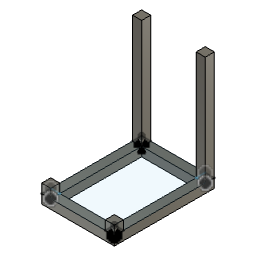
phone holder (Autodesk Fusion 360 design; units mm, degrees)
Autodesk Fusion 360 part; units mm, degrees
sketch "Sketch1" plane through (0, 0, 0) normal (0, 0, 1) x (1, 0, 0)
  line L0 (0, 0) -> (40, 0)
  line L1 (40, 0) -> (40, 55)
  line L2 (40, 55) -> (0, 55)
  line L3 (0, 55) -> (0, 0)
  line L4 (5, 5) -> (35, 5)
  line L5 (35, 5) -> (35, 50)
  line L6 (35, 50) -> (5, 50)
  line L7 (5, 50) -> (5, 5)
  dimension "d1" = 40
  dimension "d2" = 55
  dimension "d3" = 30
  dimension "d4" = 45
  constraint horizontal L0
  constraint vertical L1
  constraint horizontal L2
  constraint vertical L3
  constraint coincident L0.start L3.end
  constraint horizontal L4
  constraint vertical L5
  constraint horizontal L6
  constraint vertical L7
  measures "d1" distance of L0.start L0.end
  measures "d2" distance of L0.start L2.end
  measures "d3" distance of L4.start L4.end
  measures "d4" distance of L4.start L6.end
extrude "Extrude1" add sketch "Sketch1" along normal blind 5
sketch "Sketch2" plane through (0, 0, 5) normal (0, 0, 1) x (-1, 0, 0)
  line L0 (-5, -5) -> (-5, -50)
  line L1 (-5, -50) -> (-35, -50)
  line L2 (-35, -50) -> (-35, -5)
  line L3 (-35, -5) -> (-5, -5)
  line L4 (0, -55) -> (0, 0)
  line L5 (0, 0) -> (-40, 0)
  line L6 (-40, 0) -> (-40, -55)
  line L7 (-40, -55) -> (0, -55)
  line L8 (0, -55) -> (-5, -55)
  line L9 (-5, -55) -> (-5, -50)
  line L10 (-5, -50) -> (0, -50)
  line L11 (0, -50) -> (0, -55)
  line L12 (-35, -55) -> (-40, -55)
  line L13 (-40, -55) -> (-40, -50)
  line L14 (-40, -50) -> (-35, -50)
  line L15 (-35, -50) -> (-35, -55)
  line L16 (-35, -5) -> (-40, -5)
  line L17 (-40, -5) -> (-40, 0)
  line L18 (-40, 0) -> (-35, 0)
  line L19 (-35, 0) -> (-35, -5)
  line L20 (0, -5) -> (-5, -5)
  line L21 (-5, -5) -> (-5, 0)
  line L22 (-5, 0) -> (0, 0)
  line L23 (0, 0) -> (0, -5)
  constraint horizontal L8
  constraint vertical L9
  constraint horizontal L10
  constraint vertical L11
  constraint coincident L0.end L1.start
  constraint coincident L4.start L7.end
  constraint horizontal L12
  constraint vertical L13
  constraint horizontal L14
  constraint vertical L15
  constraint coincident L6 L13.end
  constraint coincident L7 L12.start
  constraint horizontal L16
  constraint vertical L17
  constraint horizontal L18
  constraint vertical L19
  constraint coincident L5.end L6.start
  constraint coincident L2.end L3.start
  constraint horizontal L20
  constraint vertical L21
  constraint horizontal L22
  constraint vertical L23
  constraint coincident L5 L21.end
  constraint coincident L4 L20.start
extrude "Extrude2" add sketch "Sketch2" along normal blind 5 contours L4 L5 L20 L21 L22 L23 | L5 L6 L16 L17 L18 L19
extrude "Extrude3" add sketch "Sketch2" along normal blind 60 contours L4 L7 L8 L9 L10 L11 | L6 L7 L12 L13 L14 L15
